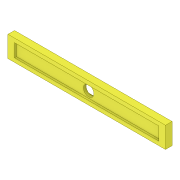
# Autodesk Inventor part: spiritLevel
Saved by Autodesk Inventor 2017 (Build 210142000, 142)
## iProperties
Created: 2017-08-08
Part Number: spiritLevel
Material: Generic
Document SubType Name: Modeling
Designer: KRosie
Density: 1 g/cm^3
Appearance: Smooth - Yellow
Author: KRosie
Autodesk Inventor part; units mm, degrees
ref_plane "YZ Plane" through (0, 0, 0) normal (1, 0, 0) x (0, 1, 0)
ref_plane "XZ Plane" through (0, 0, 0) normal (0, 1, 0) x (-1, 0, 0)
ref_plane "XY Plane" through (0, 0, 0) normal (0, 0, 1) x (1, 0, 0)
sketch "Sketch1" plane through (0, 0, 0) normal (1, 0, 0) x (0, 1, 0)
  line L0 (40, 12.5) -> (-40, 12.5)
  line L1 (-40, 12.5) -> (-40, -12.5)
  line L2 (-40, -12.5) -> (40, -12.5)
  line L3 (40, -12.5) -> (40, 12.5)
  line L4 (40, 12.5) -> (-40, -12.5) construction
  line L5 (-40, 12.5) -> (40, -12.5) construction
  point P0 (0, 0)
  dimension "d0" = 80
  dimension "d1" = 25
  constraints: 12 end point, 2 midpoint, 2 parallel, 1 horizontal, 1 perpendicular
  measures "d0" distance of L1.end L2.end
  measures "d1" distance of L0.end L1.end
extrude "Extrusion1" add sketch "Sketch1" along normal mid plane 600
sketch "Sketch2" plane through (-300, -40, 12.5) normal (0, 0, 1) x (1, 0, 0)
  circle A0 centre (300, 40) radius 20
  point P0 (300, 40)
  dimension "d4" = 40
  constraints: 1 centre point, 1 coincident
  measures "d4" diameter of A0
extrude "Extrusion2" cut sketch "Sketch2" against normal up to next
sketch "Sketch3" plane through (0, 0, 0) normal (1, 0, 0) x (0, 1, 0)
  line L0 (-25, -20) -> (25, -20)
  line L1 (25, -20) -> (25, -5)
  line L2 (25, -5) -> (-25, -5)
  line L3 (-25, -5) -> (-25, -20)
  line L4 (40, -12.5) -> (-40, -12.5) projected
  line L5 (-25, -20) -> (25, -5) construction
  line L6 (25, -20) -> (-25, -5) construction
  line L7 (20, 12.5) -> (20, -12.5) projected
  line L8 (-40, 12.5) -> (40, 12.5) projected
  line L9 (-25, 20) -> (25, 20)
  line L10 (25, 20) -> (25, 5)
  line L11 (25, 5) -> (-25, 5)
  line L12 (-25, 5) -> (-25, 20)
  line L13 (40, 12.5) -> (-40, 12.5) projected
  line L14 (-25, 20) -> (25, 5) construction
  line L15 (25, 20) -> (-25, 5) construction
  point P0 (0, -12.5)
  point P1 (20, 5)
  point P2 (0, 12.5)
  dimension "d10" = 50
  dimension "d11" = 15
  dimension "d15" = 15
  constraints: 24 end point, 6 midpoint, 4 parallel, 2 horizontal, 2 perpendicular, 1 point on line
  measures "d10" distance of L2.end L1.end
  measures "d11" distance of L1.end L0.end
  measures "d15" distance of L9.end L10.end
extrude "Extrusion3" cut sketch "Sketch3" along normal mid plane 550
body "Solid1"
